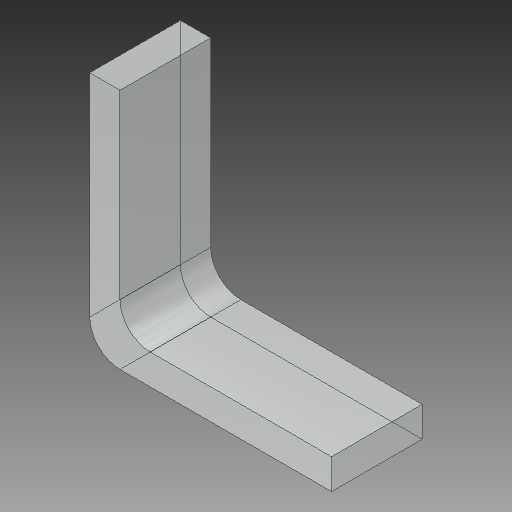
# Autodesk Inventor part: Plexi disc mount
Saved by Autodesk Inventor 2019 (Build 230136000, 136)
## iProperties
Created: 2019-02-17
Part Number: Plexi disc mount
Material: Generic
Document SubType Name: Modeling
Designer: josh
Density: 1 g/cm^3
Appearance: Clear
Mass: 11.5222 g
Surface Area: 49.768 cm^2
Volume: 11.5222 cm^3
Author: josh
Autodesk Inventor part; units mm, degrees
ref_plane "YZ Plane" through (0, 0, 0) normal (1, 0, 0) x (0, 1, 0)
ref_plane "XZ Plane" through (0, 0, 0) normal (0, 1, 0) x (-1, 0, 0)
ref_plane "XY Plane" through (0, 0, 0) normal (0, 0, 1) x (1, 0, 0)
sketch "Sketch1" plane through (0, 0, 0) normal (0, 0, 1) x (1, 0, 0)
  line L0 (6.35, 0) -> (50.8, 0)
  line L1 (50.8, 6.35) -> (12.7, 6.35)
  line L2 (0, 6.35) -> (0, 6.35)
  line L3 (6.35, 12.7) -> (6.35, 50.8)
  line L4 (0, 50.8) -> (0, 6.35)
  arc A0 (6.35, 12.7) -> (12.7, 6.35) centre (12.7, 12.7) ccw
  arc A1 (0, 6.35) -> (6.35, 0) centre (6.35, 6.35) ccw
  line L5 (50.8, 6.35) -> (50.8, 0)
  line L6 (6.35, 50.8) -> (0, 50.8)
  point P0 (0, 0)
  dimension "d4" = 6.35
  constraints: 14 end point, 4 point on circle, 4 tangent, 2 centre point, 2 parallel, 2 perpendicular, 2 point on line, 1 equal radius, 1 horizontal
  measures "d4" radius of A0
extrude "Extrusion1" add sketch "Sketch1" against normal blind 19.05
body "Solid1"
